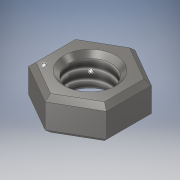
# Autodesk Inventor part: 6-32x0,25 Nut
Saved by Autodesk Inventor 2018 (Build 220112000, 112)
## iProperties
Created: 2018-05-02
Part Number: 6-32x0,25 Nut
Material: Stainless Steel
Document SubType Name: Modeling
Designer: Rich
Density: 8 g/cm^3
Appearance: Semi-Polished
Author: Rich
Autodesk Inventor part; units mm, degrees
ref_plane "YZ Plane" through (0, 0, 0) normal (1, 0, 0) x (0, 1, 0)
ref_plane "XZ Plane" through (0, 0, 0) normal (0, 1, 0) x (-1, 0, 0)
ref_plane "XY Plane" through (0, 0, 0) normal (0, 0, 1) x (1, 0, 0)
sketch "Sketch1" plane through (0, 0, 0) normal (0, 1, 0) x (-1, 0, 0)
  line L0 (0, -3.6662) -> (-3.175, -1.8331)
  line L1 (-3.175, -1.8331) -> (-3.175, 1.8331)
  line L2 (-3.175, 1.8331) -> (0, 3.6662)
  line L3 (0, 3.6662) -> (3.175, 1.8331)
  line L4 (3.175, 1.8331) -> (3.175, -1.8331)
  line L5 (3.175, -1.8331) -> (0, -3.6662)
  line L6 (0, 3.6662) -> (0, -3.6662) construction
  point P0 (0, 0)
  point P1 (0, 0)
  dimension "d0" = 6.35
  constraints: 14 end point, 1 coincident, 1 vertical, 13 other
  measures "d0" distance between parallel lines of L1 L4
extrude "Extrusion1" add sketch "Sketch1" along normal blind 2.7432
sketch "Sketch2" plane through (0, 2.7432, 0) normal (0, 1, 0) x (1, 0, 0)
  circle A0 centre (0, 0) radius 1.7526
  dimension "d3" = 3.5052
  constraints: 1 centre point, 1 coincident
  measures "d3" diameter of A0
extrude "Extrusion2" cut sketch "Sketch2" against normal blind 2.7432
chamfer "Chamfer1" distance 0.381 angle 45 14 edges at (1.5875, 2.7432, 2.7496) (-1.5875, 2.7432, 2.7496) (-3.175, 2.7432, 0) (-1.5875, 2.7432, -2.7496) (1.5875, 2.7432, -2.7496) (3.175, 2.7432, 0) (-1.7526, 2.7432, 0) (3.175, 0, 0) (1.5875, 0, 2.7496) (-1.5875, 0, 2.7496) (-3.175, 0, 0) (-1.5875, 0, -2.7496) (1.5875, 0, -2.7496) (-1.7526, 0, 0)
thread "Thread1" size "6-32 UNC" class "2B" standard "ANSI Unified Screw Threads" full length
body "Solid1"
